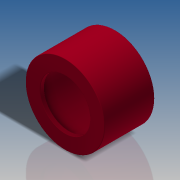
# Autodesk Inventor part: 99401-RedRubber
Saved by Autodesk Inventor 2016 SP2 (Build 200236200, 236)
## iProperties
Created: 2015-08-26
Part Number: 99401-RedRubber
Material: Rubber
Document SubType Name: Modeling
Designer: D. Kohfeld
Mass: 0.512702 g
Surface Area: 10.4616 cm^2
Volume: 0.551293 cm^3
Density: 0.93 g/cm^3
Appearance: RedRubber
Author: D. Kohfeld
Autodesk Inventor part; units mm, degrees
ref_plane "YZ Plane" through (0, 0, 0) normal (1, 0, 0) x (0, 1, 0)
ref_plane "XZ Plane" through (0, 0, 0) normal (0, 1, 0) x (-1, 0, 0)
ref_plane "XY Plane" through (0, 0, 0) normal (0, 0, 1) x (1, 0, 0)
sketch "Sketch2" plane through (0, 0, 0) normal (0, 1, 0) x (-1, 0, 0)
  line L0 (6.4, -4.8) -> (7.6, -4.8)
  line L1 (7.6, -4.8) -> (7.6, 4.8)
  line L2 (7.6, 4.8) -> (4.8, 4.8)
  line L3 (4.8, 4.8) -> (4.8, 4)
  line L4 (4.8, 4) -> (6.4, 4)
  line L5 (6.4, 4) -> (6.4, -4.8)
  line L6 (0, 4.8) -> (0, -4.8)
  point P0 (0, 0)
  point P1 (0, 0)
  dimension "d0" = 15.2
  dimension "d1" = 9.6
  dimension "d2" = 0.8
  dimension "d3" = 9.6
  dimension "d4" = 12.8
  constraints: 14 end point, 4 vertical, 3 horizontal, 2 horizontal alignment, 1 coincident, 1 midpoint
  measures "d0" diameter of L1 L6
  measures "d1" distance of L0.end L1.end
  measures "d2" distance between parallel lines of L2 L4
  measures "d3" diameter of L3 L6
  measures "d4" diameter of L5 L6
revolve "Revolution1" add sketch "Sketch2" angle 360 about axis through (0, 0, 4.8) along (0, 0, -1)
fillet "Fillet1" radius 0.1 5 edges at (4.8, 0, 4.8) (4.8, 0, 4) (7.6, 0, 4.8) (7.6, 0, -4.8) (6.4, 0, -4.8)
equation "\"d1\" = lh"
equation "\"d3\" = lh"
equation "\"lh\" = 9.6"
body "Solid1"
